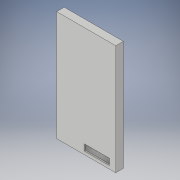
# Autodesk Inventor part: Smart Lock Box Top Correct
Saved by Autodesk Inventor 2019.3 (Build 233278000, 278)
## iProperties
Created: 2019-04-11
Part Number: Smart Lock Box Top Correct
Material: Generic
Document SubType Name: Modeling
Designer: grego
Density: 1 g/cm^3
Appearance: Default
Author: grego
Autodesk Inventor part; units mm, degrees
ref_plane "YZ Plane" through (0, 0, 0) normal (1, 0, 0) x (0, 1, 0)
ref_plane "XZ Plane" through (0, 0, 0) normal (0, 1, 0) x (-1, 0, 0)
ref_plane "XY Plane" through (0, 0, 0) normal (0, 0, 1) x (1, 0, 0)
sketch "Sketch1" plane through (0, 0, 0) normal (0, 0, 1) x (1, 0, 0)
  line L0 (-52.798, 44.3503) -> (-52.798, -78.5857)
  line L1 (-52.798, -78.5857) -> (13.242, -78.5857)
  line L2 (13.242, -78.5857) -> (13.242, 44.3503)
  line L3 (13.242, 44.3503) -> (-52.798, 44.3503)
  point P0 (0, 0)
  dimension "d0" = 122.936
  dimension "d1" = 66.04
  constraints: 8 end point, 3 perpendicular, 1 vertical
  measures "d0" distance between parallel lines of L1 L3
  measures "d1" distance between parallel lines of L2 L0
extrude "Extrusion1" add sketch "Sketch1" against normal blind 8.5
sketch "Sketch2" plane through (0, 0, -8.5) normal (0, 0, -1) x (-1, 0, 0)
  line L0 (-11.242, 42.3503) -> (50.798, 42.3503)
  line L1 (50.798, 42.3503) -> (50.798, -76.5857)
  line L2 (50.798, -76.5857) -> (-11.242, -76.5857)
  line L3 (-11.242, -76.5857) -> (-11.242, 42.3503)
  line L4 (52.798, 44.3503) -> (-13.242, 44.3503) projected
  line L5 (52.798, -78.5857) -> (52.798, 44.3503) projected
  line L6 (-13.242, 44.3503) -> (-13.242, -78.5857) projected
  line L7 (-13.242, -78.5857) -> (52.798, -78.5857) projected
  point P0 (0, 0)
  constraints: 8 end point, 2 parallel, 1 horizontal, 1 perpendicular
extrude "Extrusion2" cut sketch "Sketch2" against normal blind 7 contours L0 L1 L2 L3
sketch "Sketch3" plane through (0, 0, -1.5) normal (0, 0, -1) x (-1, 0, 0)
  line L0 (-6.162, -68.0617) -> (21.838, -68.0617)
  line L1 (21.838, -68.0617) -> (21.838, -75.0617)
  line L2 (21.838, -75.0617) -> (-6.162, -75.0617)
  line L3 (-6.162, -75.0617) -> (-6.162, -68.0617)
  line L4 (-11.242, -76.5857) -> (-11.242, 42.3503) projected
  line L5 (50.798, -76.5857) -> (-11.242, -76.5857) projected
  point P0 (0, 0)
  dimension "d10" = 5.08
  dimension "d11" = 28
  dimension "d12" = 1.524
  dimension "d13" = 7
  constraints: 8 end point, 2 parallel, 1 horizontal, 1 perpendicular
  measures "d10" distance between parallel lines of L3 L4
  measures "d11" distance between parallel lines of L1 L3
  measures "d12" distance between parallel lines of L5 L2
  measures "d13" distance between parallel lines of L2 L0
extrude "Extrusion3" cut sketch "Sketch3" against normal blind 1.5
body "Solid1"
